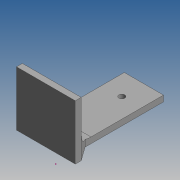
# Autodesk Inventor part: P005_supportCapteursTripod
Saved by Autodesk Inventor 2021.3 (Build 253353000, 353)
## iProperties
Created: 2021-10-05
Part Number: P005_supportCapteursTripod
Material: Générique
Document SubType Name: Modeling
Designer: gabri
Density: 1 g/cm^3
Appearance: Par défaut
Author: gabri
Autodesk Inventor part; units mm, degrees
note: some values were not read from the file. Chosen so that the rebuilt part matches the saved one: direction of "Perçage1".
ref_plane "YZ Plane" through (0, 0, 0) normal (1, 0, 0) x (0, 1, 0)
ref_plane "XZ Plane" through (0, 0, 0) normal (0, 1, 0) x (-1, 0, 0)
ref_plane "XY Plane" through (0, 0, 0) normal (0, 0, 1) x (1, 0, 0)
sketch "Esquisse2" plane through (0, 0, 0) normal (0, 0, 1) x (1, 0, 0)
  line L0 (10, 110) -> (50, 110)
  line L1 (50, 110) -> (50, 10)
  line L2 (50, 10) -> (10, 10)
  line L3 (10, 10) -> (10, 110)
  line L4 (0, 132) -> (0, -22) construction
  line L5 (-10, 0) -> (60, 0) construction
  point P0 (0, 0)
  dimension "d0" = 40
  dimension "d1" = 100
  dimension "d2" = 10
  dimension "d3" = 10
  constraints: 8 end point, 2 parallel, 1 horizontal, 1 perpendicular
  measures "d0" distance between parallel lines of L1 L3
  measures "d1" distance of L0.end L1.end
  measures "d2" distance between parallel lines of L4 L3
  measures "d3" distance between parallel lines of L5 L2
extrude "Extrusion1" add sketch "Esquisse2" along normal blind 6
sketch "Esquisse3" plane through (0, 0, 6) normal (0, 0, 1) x (1, 0, 0)
  line L0 (50, 10) -> (50, 110) construction
  line L1 (50, 110) -> (10, 110) construction
  line L2 (10, 110) -> (10, 10) construction
  line L3 (10, 10) -> (50, 10) construction
  line L4 (50, 10) -> (10, 10)
  line L5 (10, 10) -> (10, 16)
  line L6 (10, 16) -> (50, 16)
  line L7 (50, 16) -> (50, 10)
  point P0 (0, 0)
  dimension "d6" = 6
  constraints: 8 end point, 2 parallel, 1 horizontal, 1 perpendicular, 1 point on line
  measures "d6" distance between parallel lines of L3 L6
extrude "Extrusion2" add sketch "Esquisse3" along normal blind 50
sketch "Esquisse4" plane through (0, 0, 0) normal (0, 0, -1) x (-1, 0, 0)
  line L0 (-50, 10) -> (-50, 110) construction
  line L1 (-10, 10) -> (-50, 10) construction
  line L2 (-10, 110) -> (-10, 10) construction
  line L3 (-50, 110) -> (-10, 110) construction
  line L4 (-10, 110) -> (-50, 110) construction
  line L5 (-50, 110) -> (-50, 65) construction
  line L6 (-50, 65) -> (-10, 65) construction
  line L7 (-10, 65) -> (-10, 110) construction
  circle A0 centre (-30, 87.5) radius 3
  point P0 (0, 0)
  dimension "d9" = 45
  dimension "d10" = 6
  dimension "d11" = 20
  dimension "d12" = 22.5
  constraints: 8 end point, 2 parallel, 1 centre point, 1 coincident, 1 horizontal, 1 perpendicular, 1 point on line
  measures "d9" distance between parallel lines of L6 L3
  measures "d10" diameter of A0
  measures "d11" distance from line of L2 A0.centre
  measures "d12" distance from line of L3 A0.centre
hole "Perçage1" at (30, 87.5, 0) direction (0, 0, 1) diameter 6 depth 6
sketch "Esquisse5" plane through (10, 10, 0) normal (0, -1, 0) x (1, 0, 0)
  line L0 (0, 0) -> (40, 0) construction
  line L1 (40, 0) -> (40, 56) construction
  line L2 (0, 56) -> (40, 56) construction
  line L3 (0, 0) -> (0, 56) construction
  line L4 (50, 56) -> (-10, 56)
  line L5 (-10, 56) -> (-10, 0)
  line L6 (-10, 0) -> (50, 0)
  line L7 (50, 0) -> (50, 56)
  line L8 (0, 56) -> (40, 56) construction
  point P0 (-10, 0)
  dimension "d20" = 60
  dimension "d21" = 10
  constraints: 8 end point, 2 parallel, 2 point on line, 1 collinear, 1 horizontal, 1 perpendicular
  measures "d20" distance between parallel lines of L5 L7
  measures "d21" distance between parallel lines of L1 L7
extrude "Extrusion3" add sketch "Esquisse5" against normal blind 6
sketch "Esquisse6" plane through (0, 0, 0) normal (0, 0, -1) x (-1, 0, 0)
  line L0 (-10, 110) -> (-10, 16) construction
  line L1 (-50, 110) -> (-10, 110) construction
  line L2 (-50, 16) -> (-50, 110) construction
  line L3 (-60, 16) -> (-50, 16) construction
  line L4 (-60, 10) -> (-60, 16) construction
  line L5 (0, 10) -> (-60, 10) construction
  line L6 (0, 10) -> (0, 16) construction
  line L7 (-10, 16) -> (0, 16) construction
  circle A0 centre (-30, 87.5) radius 3 construction
  line L8 (0, 16) -> (-10, 30)
  line L9 (-60, 16) -> (-50, 30)
  line L10 (0, 16) -> (-10, 16)
  line L11 (-10, 16) -> (-10, 30)
  line L12 (-50, 30) -> (-50, 16)
  line L13 (-60, 16) -> (-50, 16)
  point P0 (0, 0)
  dimension "d24" = 14
  dimension "d25" = 14
  constraints: 12 end point, 4 collinear, 2 point on line
  measures "d24" vertical distance of L9.end L3.start
  measures "d25" vertical distance of L8.end L6.end
extrude "Extrusion4" add sketch "Esquisse6" against normal blind 6
sketch "Sketch7" plane through (50, 110, 6) normal (1, 0, 0) x (0, 0, -1)
  point P0 (6, -110)
fillet "Fillet1" radius 20 1 edges at (30, 16, 6)
